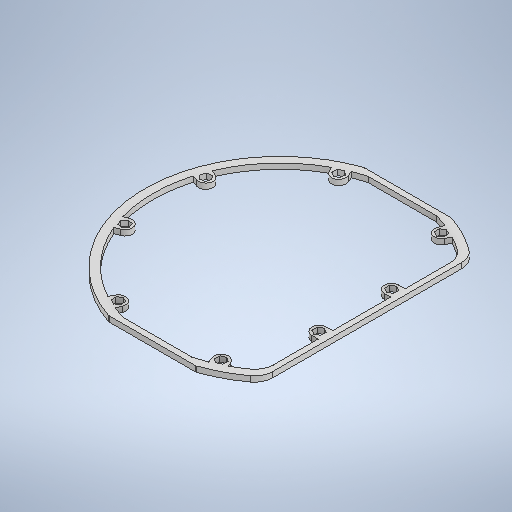
# Autodesk Inventor part: carcasa
Saved by Autodesk Inventor 2025.3 (Build 293356030, 356C)
## iProperties
Created: 2025-08-27
Part Number: carcasa
Material: Generic
Document SubType Name: Modeling
Designer: cdavi
Density: 1 g/cm^3
Appearance: Default
Author: cdavi
Autodesk Inventor part; units mm, degrees
ref_plane "YZ Plane" through (0, 0, 0) normal (1, 0, 0) x (0, 1, 0)
ref_plane "XZ Plane" through (0, 0, 0) normal (0, 1, 0) x (-1, 0, 0)
ref_plane "XY Plane" through (0, 0, 0) normal (0, 0, 1) x (1, 0, 0)
sketch "Sketch1" plane through (0, 0, 0) normal (0, 1, 0) x (-1, 0, 0)
  line L0 (18.2688, 67.5) -> (-18.2688, 67.5)
  line L1 (0, 0) -> (-48, 0) construction
  line L2 (23.7487, 70.5) -> (-23.7487, 70.5)
  line L3 (18.2688, -67.5) -> (-18.5405, -67.5)
  line L4 (23.7487, -70.5) -> (-23.7487, -70.5)
  line L5 (0, 0) -> (0, 70.5) construction
  line L6 (-45, 48.734) -> (-45, -48.734)
  line L7 (-48, 52.1177) -> (-48, -52.1177)
  arc A0 (-40.8333, -56.8563) -> (-18.5405, -67.5) centre (0, 0) ccw
  arc A1 (-43.8915, -60.1979) -> (-24.4038, -70.3897) centre (0, 0) ccw
  arc A2 (24.4038, -70.3897) -> (24.4038, 70.3897) centre (0, 0) ccw
  arc A3 (-24.4038, 70.3897) -> (-43.8915, 60.1979) centre (0, 0) ccw
  arc A4 (18.8061, -67.4265) -> (18.8061, 67.4265) centre (0, 0) ccw
  arc A5 (-18.8061, 67.4265) -> (-40.8333, 56.8563) centre (0, 0) ccw
  arc A6 (-24.4038, -70.3897) -> (-23.7487, -70.5) centre (-23.7487, -68.5) ccw
  arc A7 (23.7487, -70.5) -> (24.4038, -70.3897) centre (23.7487, -68.5) ccw
  arc A8 (18.2688, -67.5) -> (18.8061, -67.4265) centre (18.2688, -65.5) ccw
  arc A9 (18.8061, 67.4265) -> (18.2688, 67.5) centre (18.2688, 65.5) ccw
  arc A10 (24.4038, 70.3897) -> (23.7487, 70.5) centre (23.7487, 68.5) ccw
  arc A11 (-18.2688, 67.5) -> (-18.8061, 67.4265) centre (-18.2688, 65.5) ccw
  arc A12 (-23.7487, 70.5) -> (-24.4038, 70.3897) centre (-23.7487, 68.5) ccw
  arc A13 (-40.8333, 56.8563) -> (-45, 48.734) centre (-35, 48.734) ccw
  arc A14 (-43.8915, 60.1979) -> (-48, 52.1177) centre (-38, 52.1177) ccw
  arc A15 (-48, -52.1177) -> (-43.8915, -60.1979) centre (-38, -52.1177) ccw
  arc A16 (-45, -48.734) -> (-40.8333, -56.8563) centre (-35, -48.734) ccw
  point P0 (-24.0832, 70.5)
  point P1 (18.5405, -67.5)
  point P2 (24.0832, -70.5)
  point P3 (-24.0832, -70.5)
  point P4 (-48, -56.9759)
  point P5 (-45, 53.619)
  point P6 (-45, -53.619)
  point P7 (-48, 56.9759)
  point P8 (24.0832, 70.5)
  point P9 (18.5405, 67.5)
  point P10 (-18.5405, 67.5)
  dimension "d2" = 67.5
  dimension "d4" = 3
  dimension "d6" = 45
  dimension "d7" = 3
  dimension "d8" = 2
  dimension "d9" = 10
  dimension "d10" = 70
  dimension "d11" = 74.5
  dimension "d12" = 70
  dimension "d13" = 74.5
  constraints: 45 point on circle, 22 tangent, 17 centre point, 16 end point, 11 point on line, 9 equal radius, 4 symmetric about line, 3 vertical, 2 coincident, 2 horizontal, 2 midpoint, 1 parallel
  measures "d2" distance between parallel lines of L1 L0
  measures "d4" distance between parallel lines of L0 L2
  measures "d6" distance between parallel lines of L6 L5
  measures "d7" distance between parallel lines of L7 L6
  measures "d8" radius of A6
  measures "d9" radius of A13
  measures "d10" radius of A4
  measures "d11" radius of A2
  measures "d12" radius of A0
  measures "d13" radius of A1
extrude "Extrusion1" add sketch "Sketch1" along normal blind 65
sketch "Sketch2" plane through (48, 0, 52.1177) normal (1, 0, 0) x (0, 0, -1)
  line L0 (52.1177, 0) -> (52.1177, 65) construction
  line L1 (100.8516, 65) -> (3.3837, 65) projected
  line L2 (0.728, 38) -> (20.728, 38)
  line L3 (20.728, 38) -> (20.728, 26)
  line L4 (20.728, 26) -> (0.728, 26)
  line L5 (0.728, 26) -> (0.728, 38)
  line L6 (0, 0) -> (104.2353, 0) projected
  line L7 (-18.272, 0) -> (-18.272, 65) projected
  line L8 (103.5073, 38) -> (83.5073, 38)
  line L9 (83.5073, 38) -> (83.5073, 26)
  line L10 (83.5073, 26) -> (103.5073, 26)
  line L11 (103.5073, 26) -> (103.5073, 38)
  dimension "d16" = 26
  dimension "d17" = 19
  dimension "d18" = 12
  dimension "d19" = 20
  constraints: 18 end point, 4 symmetric about line, 2 parallel, 1 horizontal, 1 midpoint, 1 perpendicular
  measures "d16" distance between parallel lines of L6 L4
  measures "d17" distance between parallel lines of L5 L7
  measures "d18" distance of L2.end L3.end
  measures "d19" distance of L2.start L2.end
extrude "Extrusion2" cut sketch "Sketch2" against normal blind 5
sketch "Sketch3" plane through (48, 0, 52.1177) normal (1, 0, 0) x (0, 0, -1)
  line L0 (3.568, 49.2223) -> (17.7975, 43.9952) construction
  line L1 (2.8909, 47.379) -> (17.1204, 42.1519)
  line L2 (18.4746, 45.8385) -> (4.2452, 51.0656)
  arc A0 (4.2452, 51.0656) -> (2.8909, 47.379) centre (3.568, 49.2223) ccw
  arc A1 (17.1204, 42.1519) -> (18.4746, 45.8385) centre (17.7975, 43.9952) ccw
  arc A2 (44.4296, 11.624) -> (34.6921, 2.9774) centre (43.8866, 2.4292) ccw construction
  arc A3 (44.531, 13.3402) -> (32.9759, 3.0797) centre (43.8866, 2.4292) ccw
  arc A4 (44.3283, 9.9077) -> (36.4083, 2.8751) centre (43.8866, 2.4292) ccw
  arc A5 (44.3283, 9.9077) -> (44.531, 13.3402) centre (44.4296, 11.624) ccw
  arc A6 (32.9759, 3.0797) -> (36.4083, 2.8751) centre (34.6921, 2.9774) ccw
  line L3 (52.1177, 0) -> (52.1177, 65) construction
  line L4 (101.3444, 47.379) -> (87.1149, 42.1519)
  line L5 (85.7607, 45.8385) -> (99.9901, 51.0656)
  arc A7 (101.3444, 47.379) -> (99.9901, 51.0656) centre (100.6673, 49.2223) ccw
  arc A8 (85.7607, 45.8385) -> (87.1149, 42.1519) centre (86.4378, 43.9952) ccw
  point P0 (10.6828, 46.6088)
  constraints: 18 point on circle, 12 end point, 9 centre point, 8 tangent, 6 symmetric about line, 1 midpoint, 1 parallel, 2 other
extrude "Extrusion3" [suppressed]
extrude "Extrusion4" add sketch "Sketch1" along normal blind 3 from surface at 65 separate body contours A9 A4 A8 L3 A0 A16 L6 A13 A5 A11 L0 | A10 A2 A7 L4 A6 A1 A15 L7 A14 A3 A12 L2
sketch "Sketch5" plane through (-23.7487, 68, 70.5) normal (0, 1, 0) x (1, 0, 0)
  circle A0 centre (23.7487, 70.5) radius 8.5
  circle A1 centre (-6.2513, 70.5) radius 2.5
  line L0 (31.8727, 68) -> (40.7487, 68)
  line L1 (40.7487, 68) -> (40.7487, 73)
  line L2 (40.7487, 73) -> (31.8727, 73)
  point P0 (40.7487, 70.5)
  dimension "d26" = 17
  dimension "d27" = 5
  dimension "d31" = 5
  dimension "d32" = 17
  dimension "d47" = 30
  constraints: 6 end point, 2 centre point, 2 horizontal alignment, 2 perpendicular, 2 point on circle, 1 coincident, 1 horizontal, 1 midpoint
  measures "d26" diameter of A0
  measures "d27" diameter of A1
  measures "d31" distance between parallel lines of L2 L0
  measures "d32" distance from line of A0.centre L1
  measures "d47" distance of A0.centre A1.centre
extrude "Extrusion5" cut sketch "Sketch5" against normal through all bodies 2
sketch "Sketch6" plane through (0, 0, 0) normal (0, 1, 0) x (-1, 0, 0)
  circle A0 centre (0, 0) radius 67 construction
  arc A1 (-18.8061, 67.4265) -> (-40.8333, 56.8563) centre (0, 0) ccw projected
  arc A2 (-40.8333, 56.8563) -> (-45, 48.734) centre (-35, 48.734) ccw projected
  line L0 (-45, -48.734) -> (-45, 48.734) projected
  arc A3 (-45, -48.734) -> (-40.8333, -56.8563) centre (-35, -48.734) ccw projected
  arc A4 (-40.8333, -56.8563) -> (-18.5405, -67.5) centre (0, 0) ccw projected
  line L1 (18.2688, -67.5) -> (-18.5405, -67.5) construction
  arc A5 (18.8061, -67.4265) -> (18.8061, 67.4265) centre (0, 0) ccw projected
  line L2 (-18.2688, 67.5) -> (18.2688, 67.5) construction
  line L3 (23.7487, 70.5) -> (-23.7487, 70.5) projected
  arc A6 (-24.4038, 70.3897) -> (-43.8915, 60.1979) centre (0, 0) ccw projected
  arc A7 (-43.8915, 60.1979) -> (-48, 52.1177) centre (-38, 52.1177) ccw projected
  line L4 (-48, 52.1177) -> (-48, -52.1177) projected
  arc A8 (-48, -52.1177) -> (-43.8915, -60.1979) centre (-38, -52.1177) ccw projected
  arc A9 (-43.8915, -60.1979) -> (-24.4038, -70.3897) centre (0, 0) ccw projected
  line L5 (-23.7487, -70.5) -> (23.7487, -70.5) projected
  arc A10 (24.4038, -70.3897) -> (24.4038, 70.3897) centre (0, 0) ccw projected
  arc A11 (-17.9906, 61.4194) -> (-37.3333, 51.9829) centre (0, 0) ccw construction
  arc A12 (-37.3333, 51.9829) -> (-39, 48.734) centre (-35, 48.734) ccw construction
  line L6 (-39, 48.734) -> (-39, -48.734) construction
  arc A13 (-39, -48.734) -> (-37.3333, -51.9829) centre (-35, -48.734) ccw construction
  arc A14 (-37.3333, -51.9829) -> (-17.9906, -61.4194) centre (0, 0) ccw construction
  line L7 (-17.4284, -61.5) -> (17.4284, -61.5) construction
  line L8 (-17.4284, 61.5) -> (17.4284, 61.5) construction
  arc A15 (17.9906, -61.4194) -> (17.9906, 61.4194) centre (0, 0) ccw construction
  arc A16 (-8.124, -2.5) -> (-8.124, 2.5) centre (0, 0) ccw projected
  line L9 (0, 0) -> (63.1919, 22.2662) construction
  line L10 (0, 0) -> (74.5, 0) construction
  circle A17 centre (63.1919, 22.2662) radius 2.85 construction
  line L11 (0, 0) -> (0, -67) construction
  circle A18 centre (28.3154, 60.7226) radius 2.85 construction
  line L12 (28.3154, 60.7226) -> (0, 0) construction
  circle A19 centre (-41.5, 20) radius 2.85 construction
  circle A20 centre (-28.3154, 60.7226) radius 2.85 construction
  line L13 (-28.3154, 60.7226) -> (0, 0) construction
  arc A21 (-17.4284, 61.5) -> (-17.9906, 61.4194) centre (-17.4284, 59.5) ccw construction
  arc A22 (-17.9906, -61.4194) -> (-17.4284, -61.5) centre (-17.4284, -59.5) ccw construction
  arc A23 (17.4284, -61.5) -> (17.9906, -61.4194) centre (17.4284, -59.5) ccw construction
  arc A24 (17.9906, 61.4194) -> (17.4284, 61.5) centre (17.4284, 59.5) ccw construction
  arc A25 (-24.4038, -70.3897) -> (-23.7487, -70.5) centre (-23.7487, -68.5) ccw projected
  arc A26 (23.7487, -70.5) -> (24.4038, -70.3897) centre (23.7487, -68.5) ccw projected
  arc A27 (24.4038, 70.3897) -> (23.7487, 70.5) centre (23.7487, 68.5) ccw projected
  arc A28 (-23.7487, 70.5) -> (-24.4038, 70.3897) centre (-23.7487, 68.5) ccw projected
  circle A29 centre (63.1919, -22.2662) radius 2.85 construction
  circle A30 centre (28.3154, -60.7226) radius 2.85 construction
  circle A31 centre (-41.5, -20) radius 2.85 construction
  circle A32 centre (-28.3154, -60.7226) radius 2.85 construction
  line L14 (18.8061, 61.1746) -> (18.8061, 67.4265)
  line L15 (-18.8061, 61.1746) -> (-18.8061, 67.4265)
  line L16 (18.8061, 67.4265) -> (-18.8061, 67.4265)
  line L17 (18.8061, -61.1746) -> (18.8061, -67.4265)
  line L18 (-18.8061, -61.1746) -> (-18.8061, -67.4265)
  line L19 (18.8061, -67.4265) -> (-18.8061, -67.4265)
  circle A33 centre (63.1919, 22.2662) radius 4
  circle A34 centre (28.3154, 60.7226) radius 4
  line L20 (60.3905, 22.7899) -> (62.2448, 24.9542)
  line L21 (62.2448, 24.9542) -> (65.0462, 24.4304)
  line L22 (65.0462, 24.4304) -> (65.9934, 21.7424)
  line L23 (65.9934, 21.7424) -> (64.1391, 19.5782)
  line L24 (64.1391, 19.5782) -> (61.3376, 20.1019)
  line L25 (61.3376, 20.1019) -> (60.3905, 22.7899)
  line L26 (25.9808, 59.0879) -> (25.7324, 61.9271)
  line L27 (25.7324, 61.9271) -> (28.067, 63.5618)
  line L28 (28.067, 63.5618) -> (30.65, 62.3573)
  line L29 (30.65, 62.3573) -> (30.8984, 59.5182)
  line L30 (30.8984, 59.5182) -> (28.5638, 57.8835)
  line L31 (28.5638, 57.8835) -> (25.9808, 59.0879)
  circle A35 centre (-41.5, 20) radius 4
  line L32 (-43.9682, 18.575) -> (-43.9682, 21.425)
  line L33 (-43.9682, 21.425) -> (-41.5, 22.85)
  line L34 (-41.5, 22.85) -> (-39.0318, 21.425)
  line L35 (-39.0318, 21.425) -> (-39.0318, 18.575)
  line L36 (-39.0318, 18.575) -> (-41.5, 17.15)
  line L37 (-41.5, 17.15) -> (-43.9682, 18.575)
  line L38 (-41.5, 24) -> (-45, 24)
  line L39 (-41.5, 16) -> (-45, 16)
  circle A36 centre (-28.3154, 60.7226) radius 4
  line L40 (-28.5638, 57.8835) -> (-30.8984, 59.5182)
  line L41 (-30.8984, 59.5182) -> (-30.65, 62.3573)
  line L42 (-30.65, 62.3573) -> (-28.067, 63.5618)
  line L43 (-28.067, 63.5618) -> (-25.7324, 61.9271)
  line L44 (-25.7324, 61.9271) -> (-25.9808, 59.0879)
  line L45 (-25.9808, 59.0879) -> (-28.5638, 57.8835)
  line L46 (-31.8886, 58.9247) -> (-33.2376, 61.6057)
  circle A37 centre (63.1919, -22.2662) radius 4
  circle A38 centre (28.3154, -60.7226) radius 4
  circle A39 centre (-41.5, -20) radius 4
  line L47 (-41.5, -24) -> (-45, -24)
  line L48 (-41.5, -16) -> (-45, -16)
  circle A40 centre (-28.3154, -60.7226) radius 4
  line L49 (-31.8886, -58.9247) -> (-33.2376, -61.6057)
  line L50 (60.3905, -22.7899) -> (62.2448, -24.9542)
  line L51 (62.2448, -24.9542) -> (65.0462, -24.4304)
  line L52 (65.0462, -24.4304) -> (65.9934, -21.7424)
  line L53 (65.9934, -21.7424) -> (64.1391, -19.5782)
  line L54 (64.1391, -19.5782) -> (61.3376, -20.1019)
  line L55 (61.3376, -20.1019) -> (60.3905, -22.7899)
  line L56 (25.9808, -59.0879) -> (25.7324, -61.9271)
  line L57 (25.7324, -61.9271) -> (28.067, -63.5618)
  line L58 (28.067, -63.5618) -> (30.65, -62.3573)
  line L59 (30.65, -62.3573) -> (30.8984, -59.5182)
  line L60 (30.8984, -59.5182) -> (28.5638, -57.8835)
  line L61 (28.5638, -57.8835) -> (25.9808, -59.0879)
  line L62 (-28.5638, -57.8835) -> (-30.8984, -59.5182)
  line L63 (-30.8984, -59.5182) -> (-30.65, -62.3573)
  line L64 (-30.65, -62.3573) -> (-28.067, -63.5618)
  line L65 (-28.067, -63.5618) -> (-25.7324, -61.9271)
  line L66 (-25.7324, -61.9271) -> (-25.9808, -59.0879)
  line L67 (-25.9808, -59.0879) -> (-28.5638, -57.8835)
  line L68 (-43.9682, -18.575) -> (-43.9682, -21.425)
  line L69 (-43.9682, -21.425) -> (-41.5, -22.85)
  line L70 (-41.5, -22.85) -> (-39.0318, -21.425)
  line L71 (-39.0318, -21.425) -> (-39.0318, -18.575)
  line L72 (-39.0318, -18.575) -> (-41.5, -17.15)
  line L73 (-41.5, -17.15) -> (-43.9682, -18.575)
  line L74 (61.7506, 25.9975) -> (64.5502, 27.0789)
  line L75 (64.408, 18.4555) -> (67.2672, 19.368)
  line L76 (31.8886, 58.9247) -> (33.2376, 61.6057)
  line L77 (61.7506, -25.9975) -> (64.5502, -27.0789)
  line L78 (64.408, -18.4555) -> (67.2672, -19.368)
  line L79 (31.8886, -58.9247) -> (33.2376, -61.6057)
  line L80 (-24.6413, 62.3041) -> (-25.828, 65.0609)
  line L81 (24.6413, 62.3041) -> (25.828, 65.0609)
  line L82 (-24.6413, -62.3041) -> (-25.828, -65.0609)
  line L83 (24.6413, -62.3041) -> (25.828, -65.0609)
  point P0 (-17.713, -61.5)
  point P1 (-18.8061, 61.1746)
  point P2 (18.8061, -61.1746)
  point P3 (-18.8061, -61.1746)
  point P4 (28.3154, 60.7226)
  point P5 (28.3154, 60.7226)
  point P6 (-18.8061, -67.4265)
  point P7 (-27.1107, 64.5369)
  point P8 (-27.1107, -64.5369)
  point P9 (27.1107, -64.5369)
  point P10 (27.1107, 64.5369)
  point P11 (-45, 21.9365)
  point P12 (-45, 18.0635)
  point P13 (-32.0117, 62.2515)
  point P14 (32.0117, -62.2515)
  point P15 (66.8707, -20.6956)
  point P16 (65.0736, -25.796)
  point P17 (-32.0117, -62.2515)
  point P18 (-45, -21.9365)
  point P19 (-45, -18.0635)
  point P20 (65.0736, 25.796)
  point P21 (66.8707, 20.6956)
  point P22 (32.0117, 62.2515)
  dimension "d33" = 134
  dimension "d39" = 5.7
  dimension "d34" = 6
  dimension "d35" = 6
  dimension "d36" = 6
  dimension "d37" = 19.41
  dimension "d38" = 25
  dimension "d40" = 20
  dimension "d41" = 3.5
  dimension "d42" = 25
  dimension "d44" = 2
  dimension "d61" = 8
  dimension "d62" = 8
  dimension "d63" = 8
  dimension "d64" = 8
  constraints: 156 end point, 52 symmetric about line, 37 point on circle, 20 centre point, 16 tangent, 10 coincident, 6 perpendicular, 3 equal radius, 3 point on line, 2 parallel, 2 vertical, 93 other
  measures "d34" radial gap between concentric circles of A1 A11
  measures "d35" distance between parallel lines of L2 L8
  measures "d36" radial gap between concentric circles of A5 A15
  measures "d37" angle of L10 L9
  measures "d38" angle of L11 L12
  measures "d40" distance from line of point (-41.5, 20) L10
  measures "d41" distance from line of L0 point (-41.5, 20)
  measures "d42" angle of L11 L13
  measures "d44" radius of A21
  measures "d61" diameter of A33
  measures "d62" diameter of A34
  measures "d63" diameter of A35
  measures "d64" diameter of A36
extrude "Extrusion6" add sketch "Sketch6" against normal blind 3 separate body contours L80 A36 A1 | A36 A1 | A1 A36 | A5 A34 L81 | A36 L46 A1 | A34 A5 | A5 A34 | A5 L76 A34 | A5 A33 L74 | L38 A35 L0 | A33 A5 | A5 A33 | A35 L0 | L0 A35 | A5 L75 A33 | A35 L39 L0 | A5 A37 L78 | L48 A39 L0 | A37 A5 | A5 A37 | A39 L0 | L0 A39 | A5 L77 A37 | A39 L47 L0 | A5 A38 L79 | A38 A5 | A5 A38 | A5 L83 A38 | L49 A40 A4 | A40 A4 | A4 A40 | A40 L82 A4 | A27 A10 A26 L5 A25 A9 A8 L4 A7 A6 A28 L3
sketch "Sketch7" plane through (0, 0, 0) normal (0, 1, 0) x (1, 0, 0)
  line L0 (-29.2685, -69.2627) -> (-29.2685, 69.254)
  line L1 (-23.8326, -59.397) -> (-23.8326, -67.4265) projected
  line L2 (-79.197, 0.1644) -> (-71.0513, 0.1644)
  line L3 (-71.0513, 0.1644) -> (-71.0513, -7.8356)
  line L4 (-71.0513, 0.1644) -> (-71.0513, 8.1644)
  arc A0 (-24.4038, 70.3897) -> (-24.4038, -70.3897) centre (0, 0) ccw projected
  line L5 (-71.0513, -7.8356) -> (-74.0513, -7.8356)
  line L6 (-74.0513, -7.8356) -> (-74.0513, 8.1644)
  line L7 (-74.0513, 8.1644) -> (-71.0513, 8.1644)
  line L8 (-67.3291, -24.01) -> (-70.2482, -24.7018)
  line L9 (-70.2482, -24.7018) -> (-73.9381, -9.1331)
  line L10 (-69.174, -16.2256) -> (-67.3291, -24.01)
  line L11 (-69.174, -16.2256) -> (-71.0189, -8.4412)
  line L12 (-73.9381, -9.1331) -> (-71.0189, -8.4412)
  line L13 (-59.9771, -38.8899) -> (-62.658, -40.2363)
  line L14 (-62.658, -40.2363) -> (-69.8388, -25.9382)
  line L15 (-63.5675, -31.7409) -> (-59.9771, -38.8899)
  line L16 (-63.5675, -31.7409) -> (-67.1579, -24.5918)
  line L17 (-69.8388, -25.9382) -> (-67.1579, -24.5918)
  line L18 (-49.3918, -51.6733) -> (-51.6899, -53.6017)
  line L19 (-51.6899, -53.6017) -> (-61.9745, -41.345)
  line L20 (-54.5341, -45.545) -> (-49.3918, -51.6733)
  line L21 (-54.5341, -45.545) -> (-59.6764, -39.4166)
  line L22 (-61.9745, -41.345) -> (-59.6764, -39.4166)
  line L23 (-36.1438, -61.671) -> (-37.9352, -64.0774)
  line L24 (-37.9352, -64.0774) -> (-50.7692, -54.5228)
  line L25 (-42.5607, -56.8937) -> (-36.1438, -61.671)
  line L26 (-42.5607, -56.8937) -> (-48.9777, -52.1165)
  line L27 (-50.7692, -54.5228) -> (-48.9777, -52.1165)
  line L28 (-20.9472, -68.344) -> (-22.1354, -71.0986)
  line L29 (-22.1354, -71.0986) -> (-36.8269, -64.7613)
  line L30 (-28.2929, -65.1753) -> (-20.9472, -68.344)
  line L31 (-28.2929, -65.1753) -> (-35.6386, -62.0067)
  line L32 (-36.8269, -64.7613) -> (-35.6386, -62.0067)
  line L33 (-4.6214, -71.3325) -> (-5.1423, -74.2869)
  line L34 (-5.1423, -74.2869) -> (-20.8992, -71.5085)
  line L35 (-12.4998, -69.9433) -> (-4.6214, -71.3325)
  line L36 (-12.4998, -69.9433) -> (-20.3783, -68.5541)
  line L37 (-20.8992, -71.5085) -> (-20.3783, -68.5541)
  line L38 (11.9536, -70.4755) -> (12.1281, -73.4704)
  line L39 (12.1281, -73.4704) -> (-3.8449, -74.4007)
  line L40 (3.9672, -70.9406) -> (11.9536, -70.4755)
  line L41 (3.9672, -70.9406) -> (-4.0193, -71.4058)
  line L42 (-3.8449, -74.4007) -> (-4.0193, -71.4058)
  line L43 (27.8842, -65.8191) -> (28.7446, -68.6931)
  line L44 (28.7446, -68.6931) -> (13.4168, -73.2819)
  line L45 (20.2203, -68.1135) -> (27.8842, -65.8191)
  line L46 (20.2203, -68.1135) -> (12.5563, -70.408)
  line L47 (13.4168, -73.2819) -> (12.5563, -70.408)
  line L48 (42.3115, -57.6144) -> (43.8115, -60.2125)
  line L49 (43.8115, -60.2125) -> (29.9551, -68.2125)
  line L50 (35.3833, -61.6144) -> (42.3115, -57.6144)
  line L51 (35.3833, -61.6144) -> (28.4551, -65.6144)
  line L52 (29.9551, -68.2125) -> (28.4551, -65.6144)
  line L53 (54.4578, -46.3037) -> (56.5165, -48.4858)
  line L54 (56.5165, -48.4858) -> (44.8785, -59.4657)
  line L55 (48.6388, -51.7936) -> (54.4578, -46.3037)
  line L56 (48.6388, -51.7936) -> (42.8198, -57.2836)
  line L57 (44.8785, -59.4657) -> (42.8198, -57.2836)
  line L58 (63.6682, -32.4968) -> (66.1747, -34.1453)
  line L59 (66.1747, -34.1453) -> (57.3825, -47.5131)
  line L60 (59.2722, -39.1807) -> (63.6682, -32.4968)
  line L61 (59.2722, -39.1807) -> (54.8761, -45.8646)
  line L62 (57.3825, -47.5131) -> (54.8761, -45.8646)
  line L63 (69.4463, -16.9379) -> (72.2654, -17.964)
  line L64 (72.2654, -17.964) -> (66.7931, -32.999)
  line L65 (66.7101, -24.4554) -> (69.4463, -16.9379)
  line L66 (66.7101, -24.4554) -> (63.974, -31.973)
  line L67 (66.7931, -32.999) -> (63.974, -31.973)
  line L68 (71.4805, -0.4659) -> (74.4602, -0.8142)
  line L69 (74.4602, -0.8142) -> (72.6027, -16.706)
  line L70 (70.5518, -8.4118) -> (71.4805, -0.4659)
  line L71 (70.5518, -8.4118) -> (69.623, -16.3577)
  line L72 (72.6027, -16.706) -> (69.623, -16.3577)
  line L73 (69.6612, 16.0312) -> (72.6409, 16.3795)
  line L74 (72.6409, 16.3795) -> (74.4984, 0.4877)
  line L75 (70.5899, 8.0853) -> (69.6612, 16.0312)
  line L76 (70.5899, 8.0853) -> (71.5187, 0.1394)
  line L77 (74.4984, 0.4877) -> (71.5187, 0.1394)
  line L78 (64.0864, 31.664) -> (66.9055, 32.6901)
  line L79 (66.9055, 32.6901) -> (72.3778, 17.655)
  line L80 (66.8226, 24.1465) -> (64.0864, 31.664)
  line L81 (66.8226, 24.1465) -> (69.5588, 16.629)
  line L82 (72.3778, 17.655) -> (69.5588, 16.629)
  line L83 (55.0567, 45.5899) -> (57.5632, 47.2384)
  line L84 (57.5632, 47.2384) -> (66.3553, 33.8706)
  line L85 (59.4528, 38.906) -> (55.0567, 45.5899)
  line L86 (59.4528, 38.906) -> (63.8489, 32.2221)
  line L87 (66.3553, 33.8706) -> (63.8489, 32.2221)
  line L88 (43.0589, 57.058) -> (45.1177, 59.2401)
  line L89 (45.1177, 59.2401) -> (56.7556, 48.2602)
  line L90 (48.8779, 51.568) -> (43.0589, 57.058)
  line L91 (48.8779, 51.568) -> (54.6969, 46.0781)
  line L92 (56.7556, 48.2602) -> (54.6969, 46.0781)
  line L93 (28.7398, 65.45) -> (30.2398, 68.0481)
  line L94 (30.2398, 68.0481) -> (44.0962, 60.0481)
  line L95 (35.668, 61.45) -> (28.7398, 65.45)
  line L96 (35.668, 61.45) -> (42.5962, 57.45)
  line L97 (44.0962, 60.0481) -> (42.5962, 57.45)
  line L98 (12.8713, 70.3137) -> (13.7317, 73.1876)
  line L99 (13.7317, 73.1876) -> (29.0595, 68.5988)
  line L100 (20.5352, 68.0192) -> (12.8713, 70.3137)
  line L101 (20.5352, 68.0192) -> (28.1991, 65.7248)
  line L102 (29.0595, 68.5988) -> (28.1991, 65.7248)
  line L103 (-3.6911, 71.3867) -> (-3.5167, 74.3816)
  line L104 (-3.5167, 74.3816) -> (12.4563, 73.4513)
  line L105 (4.2954, 70.9215) -> (-3.6911, 71.3867)
  line L106 (4.2954, 70.9215) -> (12.2818, 70.4564)
  line L107 (12.4563, 73.4513) -> (12.2818, 70.4564)
  line L108 (-20.0545, 68.6112) -> (-20.5754, 71.5656)
  line L109 (-20.5754, 71.5656) -> (-4.8185, 74.344)
  line L110 (-12.176, 70.0004) -> (-20.0545, 68.6112)
  line L111 (-12.176, 70.0004) -> (-4.2976, 71.3896)
  line L112 (-4.8185, 74.344) -> (-4.2976, 71.3896)
  line L113 (-35.3368, 62.1369) -> (-36.525, 64.8916)
  line L114 (-36.525, 64.8916) -> (-21.8335, 71.2288)
  line L115 (-27.991, 65.3055) -> (-35.3368, 62.1369)
  line L116 (-27.991, 65.3055) -> (-20.6453, 68.4742)
  line L117 (-21.8335, 71.2288) -> (-20.6453, 68.4742)
  line L118 (-48.714, 52.3128) -> (-50.5055, 54.7191)
  line L119 (-50.5055, 54.7191) -> (-37.6715, 64.2737)
  line L120 (-42.297, 57.09) -> (-48.714, 52.3128)
  line L121 (-42.297, 57.09) -> (-35.88, 61.8673)
  line L122 (-37.6715, 64.2737) -> (-35.88, 61.8673)
  line L123 (-59.4651, 39.6685) -> (-61.7632, 41.5968)
  line L124 (-61.7632, 41.5968) -> (-51.4786, 53.8535)
  line L125 (-54.3228, 45.7968) -> (-59.4651, 39.6685)
  line L126 (-54.3228, 45.7968) -> (-49.1805, 51.9252)
  line L127 (-51.4786, 53.8535) -> (-49.1805, 51.9252)
  line L128 (-67.0104, 24.8856) -> (-69.6913, 26.232)
  line L129 (-69.6913, 26.232) -> (-62.5105, 40.5301)
  line L130 (-63.42, 32.0347) -> (-67.0104, 24.8856)
  line L131 (-63.42, 32.0347) -> (-59.8296, 39.1837)
  line L132 (-62.5105, 40.5301) -> (-59.8296, 39.1837)
  line L133 (-70.9431, 8.7611) -> (-73.8622, 9.453)
  line L134 (-73.8622, 9.453) -> (-70.1724, 25.0217)
  line L135 (-69.0982, 16.5455) -> (-70.9431, 8.7611)
  line L136 (-69.0982, 16.5455) -> (-67.2533, 24.3299)
  line L137 (-70.1724, 25.0217) -> (-67.2533, 24.3299)
  line L138 (-29.2685, 0.1644) -> (-79.197, 0.1644)
  arc A1 (-29.2685, 57.4953) -> (-23.8326, -59.397) centre (-6.1972, -0.0044) ccw
  arc A2 (-20.5754, 71.5656) -> (-20.8992, -71.5085) centre (-6.1972, -0.0044) ccw
  point P0 (-18.8061, -67.4265)
  dimension "d49" = 8
  dimension "d51" = 3
  dimension "d52" = 16
  dimension "d55" = 360
  constraints: 275 end point, 7 point on circle, 2 centre point, 2 perpendicular, 1 coincident, 1 horizontal, 1 point on line, 1 vertical, 278 other
  measures "d49" distance of L2.end L3.end
  measures "d51" distance of L3.end L5.end
  measures "d52" distance of L5.end L6.end
body "Solid1"
body "Solid2"
body "Solid3"
